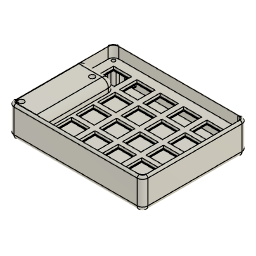
Diacritic Keypad (Autodesk Fusion 360 design; units mm, degrees)
Autodesk Fusion 360 part; units mm, degrees
sketch "Sketch1" plane through (0, 0, 0) normal (0, 0, 1) x (1, 0, 0)
  line L0 (-99.4421, 91.3159) -> (26.6579, 91.3159)
  line L1 (26.6579, 91.3159) -> (26.6579, -7.4341)
  line L2 (26.6579, -7.4341) -> (-99.4421, -7.4341)
  line L3 (-99.4421, -7.4341) -> (-99.4421, 91.3159)
  line L4 (-88.9421, 80.8159) -> (-71.8421, 80.8159)
  line L5 (-71.8421, 80.8159) -> (-71.8421, 64.5659)
  line L6 (-71.8421, 64.5659) -> (-88.9421, 64.5659)
  line L7 (-88.9421, 64.5659) -> (-88.9421, 80.8159)
  line L8 (-66.9421, 64.5659) -> (-66.9421, 80.8159)
  line L9 (-66.9421, 80.8159) -> (-49.8421, 80.8159)
  line L10 (-49.8421, 80.8159) -> (-49.8421, 64.5659)
  line L11 (-49.8421, 64.5659) -> (-66.9421, 64.5659)
  line L12 (-44.9421, 64.5659) -> (-44.9421, 80.8159)
  line L13 (-44.9421, 80.8159) -> (-27.8421, 80.8159)
  line L14 (-27.8421, 80.8159) -> (-27.8421, 64.5659)
  line L15 (-27.8421, 64.5659) -> (-44.9421, 64.5659)
  line L16 (-22.9421, 64.5659) -> (-22.9421, 80.8159)
  line L17 (-22.9421, 80.8159) -> (-5.8421, 80.8159)
  line L18 (-5.8421, 80.8159) -> (-5.8421, 64.5659)
  line L19 (-5.8421, 64.5659) -> (-22.9421, 64.5659)
  line L20 (-0.9421, 64.5659) -> (-0.9421, 80.8159)
  line L21 (-0.9421, 80.8159) -> (16.1579, 80.8159)
  line L22 (16.1579, 80.8159) -> (16.1579, 64.5659)
  line L23 (16.1579, 64.5659) -> (-0.9421, 64.5659)
  line L24 (-88.9421, 44.0659) -> (-88.9421, 60.3159)
  line L25 (-88.9421, 60.3159) -> (-71.8421, 60.3159)
  line L26 (-71.8421, 60.3159) -> (-71.8421, 44.0659)
  line L27 (-71.8421, 44.0659) -> (-88.9421, 44.0659)
  line L28 (-66.9421, 44.0659) -> (-66.9421, 60.3159)
  line L29 (-66.9421, 60.3159) -> (-49.8421, 60.3159)
  line L30 (-49.8421, 60.3159) -> (-49.8421, 44.0659)
  line L31 (-49.8421, 44.0659) -> (-66.9421, 44.0659)
  line L32 (-44.9421, 44.0659) -> (-44.9421, 60.3159)
  line L33 (-44.9421, 60.3159) -> (-27.8421, 60.3159)
  line L34 (-27.8421, 60.3159) -> (-27.8421, 44.0659)
  line L35 (-27.8421, 44.0659) -> (-44.9421, 44.0659)
  line L36 (-22.9421, 44.0659) -> (-22.9421, 60.3159)
  line L37 (-22.9421, 60.3159) -> (-5.8421, 60.3159)
  line L38 (-5.8421, 60.3159) -> (-5.8421, 44.0659)
  line L39 (-5.8421, 44.0659) -> (-22.9421, 44.0659)
  line L40 (-0.9421, 44.0659) -> (-0.9421, 60.3159)
  line L41 (-0.9421, 60.3159) -> (16.1579, 60.3159)
  line L42 (16.1579, 60.3159) -> (16.1579, 44.0659)
  line L43 (16.1579, 44.0659) -> (-0.9421, 44.0659)
  line L44 (-88.9421, 23.5659) -> (-88.9421, 39.8159)
  line L45 (-88.9421, 39.8159) -> (-71.8421, 39.8159)
  line L46 (-71.8421, 39.8159) -> (-71.8421, 23.5659)
  line L47 (-71.8421, 23.5659) -> (-88.9421, 23.5659)
  line L48 (-66.9421, 23.5659) -> (-66.9421, 39.8159)
  line L49 (-66.9421, 39.8159) -> (-49.8421, 39.8159)
  line L50 (-49.8421, 39.8159) -> (-49.8421, 23.5659)
  line L51 (-49.8421, 23.5659) -> (-66.9421, 23.5659)
  line L52 (-44.9421, 23.5659) -> (-44.9421, 39.8159)
  line L53 (-44.9421, 39.8159) -> (-27.8421, 39.8159)
  line L54 (-27.8421, 39.8159) -> (-27.8421, 23.5659)
  line L55 (-27.8421, 23.5659) -> (-44.9421, 23.5659)
  line L56 (-22.9421, 23.5659) -> (-22.9421, 39.8159)
  line L57 (-22.9421, 39.8159) -> (-5.8421, 39.8159)
  line L58 (-5.8421, 39.8159) -> (-5.8421, 23.5659)
  line L59 (-5.8421, 23.5659) -> (-22.9421, 23.5659)
  line L60 (-0.9421, 23.5659) -> (-0.9421, 39.8159)
  line L61 (-0.9421, 39.8159) -> (16.1579, 39.8159)
  line L62 (16.1579, 39.8159) -> (16.1579, 23.5659)
  line L63 (16.1579, 23.5659) -> (-0.9421, 23.5659)
  line L64 (-88.9421, 3.0659) -> (-88.9421, 19.3159)
  line L65 (-88.9421, 19.3159) -> (-71.8421, 19.3159)
  line L66 (-71.8421, 19.3159) -> (-71.8421, 3.0659)
  line L67 (-71.8421, 3.0659) -> (-88.9421, 3.0659)
  line L68 (-66.9421, 3.0659) -> (-66.9421, 19.3159)
  line L69 (-66.9421, 19.3159) -> (-49.8421, 19.3159)
  line L70 (-49.8421, 19.3159) -> (-49.8421, 3.0659)
  line L71 (-49.8421, 3.0659) -> (-66.9421, 3.0659)
  line L72 (-44.9421, 3.0659) -> (-44.9421, 19.3159)
  line L73 (-44.9421, 19.3159) -> (-27.8421, 19.3159)
  line L74 (-27.8421, 19.3159) -> (-27.8421, 3.0659)
  line L75 (-27.8421, 3.0659) -> (-44.9421, 3.0659)
  line L76 (-22.9421, 3.0659) -> (-22.9421, 19.3159)
  line L77 (-22.9421, 19.3159) -> (-5.8421, 19.3159)
  line L78 (-5.8421, 19.3159) -> (-5.8421, 3.0659)
  line L79 (-5.8421, 3.0659) -> (-22.9421, 3.0659)
  line L80 (-0.9421, 3.0659) -> (-0.9421, 19.3159)
  line L81 (-0.9421, 19.3159) -> (16.1579, 19.3159)
  line L82 (16.1579, 19.3159) -> (16.1579, 3.0659)
  line L83 (16.1579, 3.0659) -> (-0.9421, 3.0659)
  line L84 (-92.1145, 31.055) -> (-73.6145, 31.055)
  line L85 (-73.6145, 31.055) -> (-73.6145, -2.445)
  line L86 (-73.6145, -2.445) -> (-92.1145, -2.445)
  line L87 (-92.1145, -2.445) -> (-92.1145, 31.055)
  line L88 (24.6579, -5.4341) -> (-97.4421, -5.4341)
  line L89 (-97.4421, -5.4341) -> (-97.4421, 89.3159)
  line L90 (-97.4421, 89.3159) -> (24.6579, 89.3159)
  line L91 (24.6579, 89.3159) -> (24.6579, -5.4341)
  line L92 (-97.4421, 89.3159) -> (-89.4421, 89.3159)
  line L93 (-89.4421, 89.3159) -> (-89.4421, 81.3159)
  line L94 (-89.4421, 81.3159) -> (-97.4421, 81.3159)
  line L95 (-97.4421, 81.3159) -> (-97.4421, 89.3159)
  line L96 (24.6579, 89.3159) -> (16.6579, 89.3159)
  line L97 (16.6579, 89.3159) -> (16.6579, 81.3159)
  line L98 (16.6579, 81.3159) -> (24.6579, 81.3159)
  line L99 (24.6579, 81.3159) -> (24.6579, 89.3159)
  line L100 (24.6579, -5.4341) -> (16.6579, -5.4341)
  line L101 (16.6579, -5.4341) -> (16.6579, 2.5659)
  line L102 (16.6579, 2.5659) -> (24.6579, 2.5659)
  line L103 (24.6579, 2.5659) -> (24.6579, -5.4341)
  line L104 (-97.4421, -5.4341) -> (-89.4421, -5.4341)
  line L105 (-89.4421, -5.4341) -> (-89.4421, 2.5659)
  line L106 (-89.4421, 2.5659) -> (-97.4421, 2.5659)
  line L107 (-97.4421, 2.5659) -> (-97.4421, -5.4341)
  line L108 (-69.3921, 62.4409) -> (-97.4421, 62.4409)
  line L109 (-97.4421, 62.4409) -> (-97.4421, -5.4341)
  line L110 (-97.4421, -5.4341) -> (-69.3921, -5.4341)
  line L111 (-69.3921, -5.4341) -> (-69.3921, 62.4409)
  line L112 (-71.8421, 32.9465) -> (-69.3921, 32.9465) construction
  line L113 (-66.9421, 32.9465) -> (-69.3921, 32.9465) construction
  line L114 (-97.4421, 89.3159) -> (-89.4421, 81.3159) construction
  circle A0 centre (-93.4421, 85.3159) radius 2.125
  line L115 (16.6579, 81.3159) -> (24.6579, 89.3159) construction
  circle A1 centre (20.6579, 85.3159) radius 2.125
  line L116 (16.6579, 2.5659) -> (24.6579, -5.4341) construction
  line L117 (-89.4421, 2.5659) -> (-97.4421, -5.4341) construction
  circle A2 centre (-93.4421, -1.4341) radius 2.125
  circle A3 centre (20.6579, -1.4341) radius 2.125
  line L118 (-79.8732, 60.3159) -> (-79.8732, 62.4409) construction
  line L119 (-79.8732, 62.4409) -> (-79.8732, 64.5659) construction
  circle A4 centre (-93.4421, 85.3159) radius 1.625
  circle A5 centre (20.6579, 85.3159) radius 1.625
  circle A6 centre (20.6579, -1.4341) radius 1.625
  circle A7 centre (-93.4421, -1.4341) radius 1.625
  circle A8 centre (-93.4421, -1.4341) radius 2.5
  dimension "d1" = 17.1
  dimension "d2" = 16.25
  dimension "d6" = 88
  dimension "d7" = -61.5
  dimension "d8" = 4.9
  dimension "d9" = 4.25
  dimension "d10" = 10.5
  dimension "d11" = 10.5
  dimension "d12" = 10.5
  dimension "d13" = 10.5
  dimension "d14" = 18.5
  dimension "d15" = 33.5
  dimension "d16" = 2
  dimension "d21" = 8
  dimension "d22" = 8
  dimension "d23" = 8
  dimension "d24" = 8
  dimension "d25" = 8
  dimension "d26" = 8
  dimension "d27" = 8
  dimension "d28" = 8
  dimension "d76" = 4.25
  dimension "d77" = 4.25
  dimension "d78" = 4.25
  dimension "d79" = 4.25
  dimension "d106" = 3.25
  dimension "d107" = 3.25
  dimension "d108" = 3.25
  dimension "d109" = 3.25
  dimension "d112" = 5
  constraint horizontal L0
  constraint vertical L1
  constraint horizontal L2
  constraint vertical L3
  constraint horizontal L4
  constraint vertical L5
  constraint horizontal L6
  constraint vertical L7
  constraint horizontal L84
  constraint vertical L85
  constraint horizontal L86
  constraint vertical L87
  constraint horizontal L92
  constraint vertical L93
  constraint horizontal L94
  constraint vertical L95
  constraint horizontal L96
  constraint vertical L97
  constraint horizontal L98
  constraint vertical L99
  constraint horizontal L100
  constraint vertical L101
  constraint horizontal L102
  constraint vertical L103
  constraint horizontal L104
  constraint vertical L105
  constraint horizontal L106
  constraint vertical L107
  constraint horizontal L108
  constraint vertical L109
  constraint horizontal L110
  constraint vertical L111
  constraint coincident L46 L112.start
  constraint coincident L111 L112.end
  constraint perpendicular L111 L112
  constraint coincident L48 L113.start
  constraint perpendicular L111 L113
  constraint equal L112 L113
  constraint midpoint L114 A0.centre
  constraint midpoint L115 A1.centre
  constraint midpoint L117 A2.centre
  constraint midpoint L116 A3.centre
  constraint coincident L25 L118.start
  constraint coincident L108 L118.end
  constraint perpendicular L108 L118
  constraint coincident L6 L119.end
  constraint perpendicular L6 L119
  constraint equal L118 L119
  constraint concentric A0 A4
  constraint concentric A1 A5
  constraint concentric A3 A6
  constraint concentric A2 A7
  constraint concentric A2 A8
  measures "d1" distance of L4.start L4.end
  measures "d2" distance of L4.start L6.end
  measures "d8" distance of L5 L8
  measures "d9" distance of L6 L25
  measures "d10" distance of L0 L4
  measures "d11" distance of L3 L7
  measures "d12" distance of L1 L22
  measures "d13" distance of L2 L83
  measures "d14" distance of L84.start L84.end
  measures "d15" distance of L84.start L86.end
  measures "d21" distance of L89.end L92.end
  measures "d22" distance of L89.end L94.end
  measures "d23" distance of L90.end L96.end
  measures "d24" distance of L90.end L98.end
  measures "d25" distance of L88.start L100.end
  measures "d26" distance of L88.start L102.end
  measures "d27" distance of L88.end L104.end
  measures "d28" distance of L88.end L106.end
  measures "d76" diameter of A0
  measures "d77" diameter of A1
  measures "d78" diameter of A2
  measures "d79" diameter of A3
  measures "d106" diameter of A4
  measures "d107" diameter of A5
  measures "d108" diameter of A6
  measures "d109" diameter of A7
  measures "d112" diameter of A8
extrude "Extrude1" add sketch "Sketch1" against normal blind 2 contours L0 L1 L2 L3 | L4 L5 L6 L7 | L8 L9 L10 L11 | L12 L13 L14 L15 | L16 L17 L18 L19 | L20 L21 L22 L23 | L24 L25 L26 L27 | L28 L29 L30 L31 | L32 L33 L34 L35 | L36 L37 L38 L39 | L40 L41 L42 L43 | L44 L47 L64 L65 L67 L84 L85 L86 L87 L105 L106 | L44 L47 L84 L85 | L44 L45 L46 L47 L65 L66 L67 L84 L85 L86 L87 L88 L89 L105 L106 L108 L109 L110 L111 | L44 L45 L46 L47 L84 L85 | L64 L65 L67 L85 | L65 L66 L67 L85 | L86 L87 L105 L106 A8 | L86 L87 L88 L89 L104 L105 L106 L107 L109 L110 A8 | L86 L87 A2 A8 | L86 L87 A2 A8 | L86 L87 A2 A7 | L86 L87 A2 A7 | L88 L89 L90 L91 L93 L94 L97 L98 L101 L102 L108 L111 | L87 A7 | L87 A7 | L89 L90 L92 L93 L94 L95 | L88 L91 L100 L101 L102 L103 | L90 L91 L96 L97 L98 L99 | L48 L49 L50 L51 | L52 L53 L54 L55 | L56 L57 L58 L59 | L60 L61 L62 L63 | L68 L69 L70 L71 | L72 L73 L74 L75 | L76 L77 L78 L79 | L80 L81 L82 L83 | A0 | A1 | A3 | A4 | A5 | A6 makes body 1
extrude "Extrude2" add sketch "Sketch1" along normal blind 28 contours L0 L1 L2 L3 bodies 1
extrude "Extrude3" add sketch "Sketch1" along normal blind 14.5 contours L86 L87 L105 L106 A8 | L86 L87 L88 L89 L104 L105 L106 L107 L109 L110 A8 | L86 L87 A2 A8 | L86 L87 A2 A8 | L89 L90 L92 L93 L94 L95 | L88 L91 L100 L101 L102 L103 | L90 L91 L96 L97 L98 L99 bodies 1
extrude "Extrude4" add sketch "Sketch1" along normal blind 2.5 from surface at 14.5 separate body contours L44 L47 L64 L65 L67 L84 L85 L86 L87 L105 L106 | L44 L47 L84 L85 | L44 L45 L46 L47 L65 L66 L67 L84 L85 L86 L87 L88 L89 L105 L106 L108 L109 L110 L111 | L44 L45 L46 L47 L84 L85 | L64 L65 L67 L85 | L65 L66 L67 L85 | L86 L87 L105 L106 A8 | L86 L87 L88 L89 L104 L105 L106 L107 L109 L110 A8 | L86 L87 A2 A8 | L86 L87 A2 A8 | L86 L87 A2 A7 | L86 L87 A2 A7 | L88 L89 L90 L91 L93 L94 L97 L98 L101 L102 L108 L111 | L87 A7 | L87 A7 | L89 L90 L92 L93 L94 L95 | L88 L91 L100 L101 L102 L103 | L90 L91 L96 L97 L98 L99 | A0 | A1 | A3 | A4 | A5 | A6 makes body 2
extrude "Extrude5" cut 1 faces at (-16.0421, -6.7674, 28) along direction (0, 0, -1) blind 0.4 on bodies 1 bodies 1
extrude "Extrude7" add sketch "Sketch1" along normal blind 10 from surface at 17 contours L24 L25 L26 L27 | L44 L47 L64 L65 L67 L84 L85 L86 L87 L105 L106 | L44 L47 L84 L85 | L44 L45 L46 L47 L65 L66 L67 L84 L85 L86 L87 L88 L89 L105 L106 L108 L109 L110 L111 | L44 L45 L46 L47 L84 L85 | L64 L65 L67 L85 | L65 L66 L67 L85 | L86 L87 L105 L106 A8 | L86 L87 L88 L89 L104 L105 L106 L107 L109 L110 A8 | L86 L87 A2 A8 | L86 L87 A2 A8 | L86 L87 A2 A7 | L86 L87 A2 A7 | L87 A7 | L87 A7 bodies 2
extrude "Extrude8" cut 1 faces at (-88.0921, -5.4341, 19.5) along direction (0, 1, 0) blind 0.3 on bodies 2 bodies 2
extrude "Extrude9" cut 1 faces at (24.6579, 57.8326, 15.3333) along direction (-1, 0, 0) blind 0.3 on bodies 2 bodies 2
extrude "Extrude10" cut 1 faces at (-56.8421, 89.3159, 15.3333) along direction (0, -1, 0) blind 0.3 on bodies 2 bodies 2
extrude "Extrude11" cut 1 faces at (-97.4421, 17.3909, 19.5) along direction (1, 0, 0) blind 0.3 on bodies 2 bodies 2
extrude "Extrude19" cut sketch "Sketch1" along normal blind 18 contours L87 A7 | L87 A7 | A4 | A5 | A6 bodies 2
extrude "Extrude20" cut sketch "Sketch1" along normal blind 15.5 from surface at 18 contours L86 L87 A2 A8 | L86 L87 A2 A8 | L86 L87 A2 A7 | L86 L87 A2 A7 | L87 A7 | L87 A7 bodies 2
fillet "Fillet1" radius 5 12 edges at (-99.4421, -7.4341, 12.8) (-99.4421, 91.3159, 12.8) (26.6579, 91.3159, 12.8) (26.6579, -7.4341, 12.8) (24.6579, -5.4341, 21.05) (-97.4421, -5.4341, 21.05) (-97.4421, 89.3159, 21.05) (24.6579, 89.3159, 21.05) (-97.1421, -5.1341, 20.75) (-97.1421, 89.0159, 15.75) (24.3579, 89.0159, 15.75) (24.3579, -5.1341, 15.75) on bodies 1 2
fillet "Fillet2" radius 5 8 edges at (25.1934, -5.9696, -2) (-36.3921, -7.4341, -2) (-97.9776, -5.9696, -2) (-99.4421, 41.9409, -2) (-97.9776, 89.8515, -2) (-36.3921, 91.3159, -2) (25.1934, 89.8515, -2) (26.6579, 41.9409, -2) on bodies 1
fillet "Fillet3" radius 2 8 edges at (-36.3921, 91.3159, 27.6) (25.1934, 89.8515, 27.6) (26.6579, 41.9409, 27.6) (25.1934, -5.9696, 27.6) (-36.3921, -7.4341, 27.6) (-97.9776, -5.9696, 27.6) (-99.4421, 41.9409, 27.6) (-97.9776, 89.8515, 27.6) on bodies 1
fillet "Fillet4" radius 6 3 edges at (-83.2671, 62.4409, 27) (-69.3921, 28.6534, 27) (-69.3921, 62.4409, 22) on bodies 2
fillet "Fillet5" radius 2.5 12 edges at (-97.4421, 81.3159, 7.25) (-89.4421, 81.3159, 7.25) (-89.4421, 89.3159, 7.25) (16.6579, 89.3159, 7.25) (16.6579, 81.3159, 7.25) (24.6579, 81.3159, 7.25) (-89.4421, -5.4341, 7.25) (-89.4421, 2.5659, 7.25) (-97.4421, 2.5659, 7.25) (16.6579, -5.4341, 7.25) (16.6579, 2.5659, 7.25) (24.6579, 2.5659, 7.25) on bodies 1
extrude "Extrude12" add 4 faces at (-94, -2.432, 0) (21.3662, 84.3524, 0) (20.0197, -1.7414, 0) (-92.5065, 85.7665, 0) along direction (0, 0, 1) blind 4 on bodies 1 bodies 1
sketch "Sketch2" plane through (0, 0, 14.5) normal (0, 0, -1) x (1, 0, 0)
  line L0 (-27.8421, -19.3159) -> (-44.9421, -19.3159)
  line L1 (-44.9421, -19.3159) -> (-44.9421, -3.0659)
  line L2 (-44.9421, -3.0659) -> (-27.8421, -3.0659)
  line L3 (-27.8421, -3.0659) -> (-27.8421, -19.3159)
  line L4 (-5.8421, -19.3159) -> (-22.9421, -19.3159)
  line L5 (-22.9421, -19.3159) -> (-22.9421, -3.0659)
  line L6 (-22.9421, -3.0659) -> (-5.8421, -3.0659)
  line L7 (-5.8421, -3.0659) -> (-5.8421, -19.3159)
  line L8 (16.1579, -19.3159) -> (-0.9421, -19.3159)
  line L9 (-0.9421, -19.3159) -> (-0.9421, -3.0659)
  line L10 (-0.9421, -3.0659) -> (16.1579, -3.0659)
  line L11 (16.1579, -3.0659) -> (16.1579, -19.3159)
  line L12 (-71.8421, -64.5659) -> (-71.8421, -80.8159)
  line L13 (-71.8421, -80.8159) -> (-88.9421, -80.8159)
  line L14 (-88.9421, -80.8159) -> (-88.9421, -64.5659)
  line L15 (-88.9421, -64.5659) -> (-71.8421, -64.5659)
  line L16 (-49.8421, -80.8159) -> (-66.9421, -80.8159)
  line L17 (-66.9421, -80.8159) -> (-66.9421, -64.5659)
  line L18 (-66.9421, -64.5659) -> (-49.8421, -64.5659)
  line L19 (-49.8421, -64.5659) -> (-49.8421, -80.8159)
  line L20 (-5.8421, -80.8159) -> (-22.9421, -80.8159)
  line L21 (-22.9421, -80.8159) -> (-22.9421, -64.5659)
  line L22 (-22.9421, -64.5659) -> (-5.8421, -64.5659)
  line L23 (-5.8421, -64.5659) -> (-5.8421, -80.8159)
  line L24 (-27.8421, -80.8159) -> (-44.9421, -80.8159)
  line L25 (-44.9421, -80.8159) -> (-44.9421, -64.5659)
  line L26 (-44.9421, -64.5659) -> (-27.8421, -64.5659)
  line L27 (-27.8421, -64.5659) -> (-27.8421, -80.8159)
  line L28 (-49.8421, -39.8159) -> (-66.9421, -39.8159)
  line L29 (-66.9421, -39.8159) -> (-66.9421, -23.5659)
  line L30 (-66.9421, -23.5659) -> (-49.8421, -23.5659)
  line L31 (-49.8421, -23.5659) -> (-49.8421, -39.8159)
  line L32 (-5.8421, -60.3159) -> (-22.9421, -60.3159)
  line L33 (-22.9421, -60.3159) -> (-22.9421, -44.0659)
  line L34 (-22.9421, -44.0659) -> (-5.8421, -44.0659)
  line L35 (-5.8421, -44.0659) -> (-5.8421, -60.3159)
  line L36 (-49.8421, -60.3159) -> (-66.9421, -60.3159)
  line L37 (-66.9421, -60.3159) -> (-66.9421, -44.0659)
  line L38 (-66.9421, -44.0659) -> (-49.8421, -44.0659)
  line L39 (-49.8421, -44.0659) -> (-49.8421, -60.3159)
  line L40 (16.1579, -39.8159) -> (-0.9421, -39.8159)
  line L41 (-0.9421, -39.8159) -> (-0.9421, -23.5659)
  line L42 (-0.9421, -23.5659) -> (16.1579, -23.5659)
  line L43 (16.1579, -23.5659) -> (16.1579, -39.8159)
  line L44 (-49.8421, -19.3159) -> (-66.9421, -19.3159)
  line L45 (-66.9421, -19.3159) -> (-66.9421, -3.0659)
  line L46 (-66.9421, -3.0659) -> (-49.8421, -3.0659)
  line L47 (-49.8421, -3.0659) -> (-49.8421, -19.3159)
  line L48 (-5.8421, -39.8159) -> (-22.9421, -39.8159)
  line L49 (-22.9421, -39.8159) -> (-22.9421, -23.5659)
  line L50 (-22.9421, -23.5659) -> (-5.8421, -23.5659)
  line L51 (-5.8421, -23.5659) -> (-5.8421, -39.8159)
  line L52 (-27.8421, -60.3159) -> (-44.9421, -60.3159)
  line L53 (-44.9421, -60.3159) -> (-44.9421, -44.0659)
  line L54 (-44.9421, -44.0659) -> (-27.8421, -44.0659)
  line L55 (-27.8421, -44.0659) -> (-27.8421, -60.3159)
  line L56 (-71.8421, -60.3159) -> (-88.9421, -60.3159)
  line L57 (-88.9421, -60.3159) -> (-88.9421, -44.0659)
  line L58 (-88.9421, -44.0659) -> (-71.8421, -44.0659)
  line L59 (-71.8421, -44.0659) -> (-71.8421, -60.3159)
  line L60 (-27.8421, -39.8159) -> (-44.9421, -39.8159)
  line L61 (-44.9421, -39.8159) -> (-44.9421, -23.5659)
  line L62 (-44.9421, -23.5659) -> (-27.8421, -23.5659)
  line L63 (-27.8421, -23.5659) -> (-27.8421, -39.8159)
  line L64 (16.1579, -80.8159) -> (-0.9421, -80.8159)
  line L65 (-0.9421, -80.8159) -> (-0.9421, -64.5659)
  line L66 (-0.9421, -64.5659) -> (16.1579, -64.5659)
  line L67 (16.1579, -64.5659) -> (16.1579, -80.8159)
  line L68 (16.1579, -60.3159) -> (-0.9421, -60.3159)
  line L69 (-0.9421, -60.3159) -> (-0.9421, -44.0659)
  line L70 (-0.9421, -44.0659) -> (16.1579, -44.0659)
  line L71 (16.1579, -44.0659) -> (16.1579, -60.3159)
  line L72 (-50.4671, -18.6909) -> (-66.3171, -18.6909)
  line L73 (-66.3171, -18.6909) -> (-66.3171, -3.6909)
  line L74 (-66.3171, -3.6909) -> (-50.4671, -3.6909)
  line L75 (-50.4671, -3.6909) -> (-50.4671, -18.6909)
  line L76 (-28.4671, -3.6909) -> (-28.4671, -18.6909)
  line L77 (-28.4671, -18.6909) -> (-44.3171, -18.6909)
  line L78 (-44.3171, -18.6909) -> (-44.3171, -3.6909)
  line L79 (-44.3171, -3.6909) -> (-28.4671, -3.6909)
  line L80 (-6.4671, -18.6909) -> (-22.3171, -18.6909)
  line L81 (-22.3171, -18.6909) -> (-22.3171, -3.6909)
  line L82 (-22.3171, -3.6909) -> (-6.4671, -3.6909)
  line L83 (-6.4671, -3.6909) -> (-6.4671, -18.6909)
  line L84 (-0.3171, -3.6909) -> (15.5329, -3.6909)
  line L85 (15.5329, -3.6909) -> (15.5329, -18.6909)
  line L86 (15.5329, -18.6909) -> (-0.3171, -18.6909)
  line L87 (-0.3171, -18.6909) -> (-0.3171, -3.6909)
  line L88 (-50.4671, -39.1909) -> (-66.3171, -39.1909)
  line L89 (-66.3171, -39.1909) -> (-66.3171, -24.1909)
  line L90 (-66.3171, -24.1909) -> (-50.4671, -24.1909)
  line L91 (-50.4671, -24.1909) -> (-50.4671, -39.1909)
  line L92 (-28.4671, -24.1909) -> (-28.4671, -39.1909)
  line L93 (-28.4671, -39.1909) -> (-44.3171, -39.1909)
  line L94 (-44.3171, -39.1909) -> (-44.3171, -24.1909)
  line L95 (-44.3171, -24.1909) -> (-28.4671, -24.1909)
  line L96 (-6.4671, -39.1909) -> (-22.3171, -39.1909)
  line L97 (-22.3171, -39.1909) -> (-22.3171, -24.1909)
  line L98 (-22.3171, -24.1909) -> (-6.4671, -24.1909)
  line L99 (-6.4671, -24.1909) -> (-6.4671, -39.1909)
  line L100 (15.5329, -39.1909) -> (-0.3171, -39.1909)
  line L101 (-0.3171, -39.1909) -> (-0.3171, -24.1909)
  line L102 (-0.3171, -24.1909) -> (15.5329, -24.1909)
  line L103 (15.5329, -24.1909) -> (15.5329, -39.1909)
  line L104 (15.5329, -44.6909) -> (15.5329, -59.6909)
  line L105 (15.5329, -59.6909) -> (-0.3171, -59.6909)
  line L106 (-0.3171, -59.6909) -> (-0.3171, -44.6909)
  line L107 (-0.3171, -44.6909) -> (15.5329, -44.6909)
  line L108 (-6.4671, -59.6909) -> (-22.3171, -59.6909)
  line L109 (-22.3171, -59.6909) -> (-22.3171, -44.6909)
  line L110 (-22.3171, -44.6909) -> (-6.4671, -44.6909)
  line L111 (-6.4671, -44.6909) -> (-6.4671, -59.6909)
  line L112 (-44.3171, -59.6909) -> (-44.3171, -44.6909)
  line L113 (-44.3171, -44.6909) -> (-28.4671, -44.6909)
  line L114 (-28.4671, -44.6909) -> (-28.4671, -59.6909)
  line L115 (-28.4671, -59.6909) -> (-44.3171, -59.6909)
  line L116 (-66.3171, -59.6909) -> (-66.3171, -44.6909)
  line L117 (-66.3171, -44.6909) -> (-50.4671, -44.6909)
  line L118 (-50.4671, -44.6909) -> (-50.4671, -59.6909)
  line L119 (-50.4671, -59.6909) -> (-66.3171, -59.6909)
  line L120 (-88.3171, -59.6909) -> (-88.3171, -44.6909)
  line L121 (-88.3171, -44.6909) -> (-72.4671, -44.6909)
  line L122 (-72.4671, -44.6909) -> (-72.4671, -59.6909)
  line L123 (-72.4671, -59.6909) -> (-88.3171, -59.6909)
  line L124 (-88.3171, -80.1909) -> (-88.3171, -65.1909)
  line L125 (-88.3171, -65.1909) -> (-72.4671, -65.1909)
  line L126 (-72.4671, -65.1909) -> (-72.4671, -80.1909)
  line L127 (-72.4671, -80.1909) -> (-88.3171, -80.1909)
  line L128 (-50.4671, -65.1909) -> (-50.4671, -80.1909)
  line L129 (-50.4671, -80.1909) -> (-66.3171, -80.1909)
  line L130 (-66.3171, -80.1909) -> (-66.3171, -65.1909)
  line L131 (-66.3171, -65.1909) -> (-50.4671, -65.1909)
  line L132 (-28.4671, -65.1909) -> (-28.4671, -80.1909)
  line L133 (-28.4671, -80.1909) -> (-44.3171, -80.1909)
  line L134 (-44.3171, -80.1909) -> (-44.3171, -65.1909)
  line L135 (-44.3171, -65.1909) -> (-28.4671, -65.1909)
  line L136 (-6.4671, -80.1909) -> (-22.3171, -80.1909)
  line L137 (-22.3171, -80.1909) -> (-22.3171, -65.1909)
  line L138 (-22.3171, -65.1909) -> (-6.4671, -65.1909)
  line L139 (-6.4671, -65.1909) -> (-6.4671, -80.1909)
  line L140 (15.5329, -65.1909) -> (15.5329, -80.1909)
  line L141 (15.5329, -80.1909) -> (-0.3171, -80.1909)
  line L142 (-0.3171, -80.1909) -> (-0.3171, -65.1909)
  line L143 (-0.3171, -65.1909) -> (15.5329, -65.1909)
  arc A0 (24.3579, 0.1341) -> (19.3579, 5.1341) centre (19.3579, 0.1341) ccw
  line L144 (19.3579, 5.1341) -> (-92.1421, 5.1341)
  arc A1 (-92.1421, 5.1341) -> (-97.1421, 0.1341) centre (-92.1421, 0.1341) ccw
  line L145 (-97.1421, 0.1341) -> (-97.1421, -84.0159)
  arc A2 (-97.1421, -84.0159) -> (-92.1421, -89.0159) centre (-92.1421, -84.0159) ccw
  line L146 (-92.1421, -89.0159) -> (19.3579, -89.0159)
  arc A3 (19.3579, -89.0159) -> (24.3579, -84.0159) centre (19.3579, -84.0159) ccw
  line L147 (24.3579, -84.0159) -> (24.3579, 0.1341)
  circle A4 centre (-93.4421, 1.4341) radius 1.625
  circle A5 centre (-93.4421, -85.3159) radius 1.625
  circle A6 centre (20.6579, 1.4341) radius 1.625
  circle A7 centre (20.6579, -85.3159) radius 1.625
  dimension "d36" = 0.625
  dimension "d37" = 0.625
  dimension "d39" = 0.625
  dimension "d40" = 0.625
  dimension "d41" = 0.625
  dimension "d42" = 0.625
  dimension "d43" = 0.625
  dimension "d44" = 0.625
  dimension "d45" = 0.625
  dimension "d46" = 0.625
  dimension "d47" = 0.625
  dimension "d48" = 0.625
  dimension "d49" = 0.625
  dimension "d50" = 0.625
  dimension "d51" = 0.625
  dimension "d52" = 0.625
  dimension "d53" = 0.625
  dimension "d54" = 0.625
extrude "Extrude6" add sketch "Sketch2" along normal blind 0.6 contours L0 L1 L2 L3 | L4 L5 L6 L7 | L8 L9 L10 L11 | L12 L13 L14 L15 | L16 L17 L18 L19 | L20 L21 L22 L23 | L24 L25 L26 L27 | L28 L29 L30 L31 | L32 L33 L34 L35 | L36 L37 L38 L39 | L40 L41 L42 L43 | L44 L45 L46 L47 | L48 L49 L50 L51 | L52 L53 L54 L55 | L56 L57 L58 L59 | L60 L61 L62 L63 | L64 L65 L66 L67 | L68 L69 L70 L71 | A0 L144 A1 L145 A2 L146 A3 L147 bodies 2
move_body "Move1" bodies 2 to x (1, 0, 0) y (0, 1, 0) z (0, 0, 1) at (0, 0, 0.6)
extrude "Extrude13" add 1 faces at (-77.5421, 49.4826, 17.6) along direction (0, 0, -1) blind 3.1 on bodies 2 bodies 2
sketch "Sketch3" plane through (-97.4421, 0, 0) normal (1, 0, 0) x (0, 1, 0)
  line L0 (5.0659, 14.5) -> (5.0659, 0)
  line L1 (5.0659, 0) -> (78.8159, 0)
  line L2 (78.8159, 0) -> (78.8159, 14.5)
  line L3 (78.8159, 14.5) -> (84.3159, 14.5)
  line L4 (84.3159, 14.5) -> (84.3159, 27.6)
  line L5 (84.3159, 27.6) -> (-0.4341, 27.6)
  line L6 (-0.4341, 27.6) -> (-0.4341, 14.5)
  line L7 (-0.4341, 14.5) -> (5.0659, 14.5)
  line L8 (55.3537, 12.9074) -> (76.1037, 12.9074)
  line L9 (76.1037, 12.9074) -> (76.1037, 1.0574)
  line L10 (76.1037, 1.0574) -> (55.3537, 1.0574)
  line L11 (55.3537, 1.0574) -> (55.3537, 12.9074)
  dimension "d86" = 20.75
  dimension "d87" = 11.85
  constraint horizontal L8
  constraint vertical L9
  constraint horizontal L10
  constraint vertical L11
  measures "d86" distance of L8.start L8.end
  measures "d87" distance of L8.start L10.end
extrude "Extrude14" cut sketch "Sketch3" against normal blind 5 contours L8 L9 L10 L11 bodies 1
sketch "Sketch4" plane through (0, 89.3159, 0) normal (0, -1, 0) x (1, 0, 0)
  line L0 (14.1579, 0) -> (14.1579, 14.5)
  line L1 (14.1579, 14.5) -> (19.6579, 14.5)
  line L2 (19.6579, 14.5) -> (19.6579, 27.6)
  line L3 (19.6579, 27.6) -> (-92.4421, 27.6)
  line L4 (-92.4421, 27.6) -> (-92.4421, 14.5)
  line L5 (-92.4421, 14.5) -> (-86.9421, 14.5)
  line L6 (-86.9421, 14.5) -> (-86.9421, 0)
  line L7 (-86.9421, 0) -> (14.1579, 0)
  line L8 (-86.5962, 7.1262) -> (-76.0962, 7.1262)
  line L9 (-76.0962, 7.1262) -> (-76.0962, 1.1262)
  line L10 (-76.0962, 1.1262) -> (-86.5962, 1.1262)
  line L11 (-86.5962, 1.1262) -> (-86.5962, 7.1262)
  dimension "d90" = 10.5
  dimension "d91" = 6
  constraint horizontal L8
  constraint vertical L9
  constraint horizontal L10
  constraint vertical L11
  measures "d90" distance of L8.start L8.end
  measures "d91" distance of L8.start L10.end
extrude "Extrude15" cut sketch "Sketch4" against normal blind 7 contours L8 L9 L10 L11 bodies 1
fillet "Fillet6" radius 2.25 4 edges at (-76.0962, 90.1337, 1.1262) (-76.0962, 90.3159, 7.1262) (-86.5962, 90.3159, 7.1262) (-86.5962, 90.1337, 1.1262) on bodies 1
sketch "Sketch5" plane through (0, 0, 27.6) normal (0, 0, 1) x (-1, 0, 0)
  line L0 (75.3921, -56.4409) -> (97.1421, -56.4409)
  line L1 (97.1421, -56.4409) -> (97.1421, 0.1341)
  arc A0 (97.1421, 0.1341) -> (92.1421, 5.1341) centre (92.1421, 0.1341) ccw
  line L2 (92.1421, 5.1341) -> (75.3921, 5.1341)
  line L3 (75.3921, 5.1341) -> (75.3921, -56.4409)
  circle A1 centre (80.3921, -52.1909) radius 2.425
  circle A2 centre (80.3921, -52.1909) radius 3.125
  line L4 (22.9421, -60.3159) -> (5.8421, -60.3159)
  line L5 (5.8421, -60.3159) -> (5.8421, -44.0659)
  line L6 (5.8421, -44.0659) -> (22.9421, -44.0659)
  line L7 (22.9421, -44.0659) -> (22.9421, -60.3159)
  line L8 (44.9421, -60.3159) -> (27.8421, -60.3159)
  line L9 (27.8421, -60.3159) -> (27.8421, -44.0659)
  line L10 (27.8421, -44.0659) -> (44.9421, -44.0659)
  line L11 (44.9421, -44.0659) -> (44.9421, -60.3159)
  line L12 (66.9421, -60.3159) -> (49.8421, -60.3159)
  line L13 (49.8421, -60.3159) -> (49.8421, -44.0659)
  line L14 (49.8421, -44.0659) -> (66.9421, -44.0659)
  line L15 (66.9421, -44.0659) -> (66.9421, -60.3159)
  line L16 (0.9421, -80.8159) -> (-16.1579, -80.8159)
  line L17 (-16.1579, -80.8159) -> (-16.1579, -64.5659)
  line L18 (-16.1579, -64.5659) -> (0.9421, -64.5659)
  line L19 (0.9421, -64.5659) -> (0.9421, -80.8159)
  line L20 (66.9421, -39.8159) -> (49.8421, -39.8159)
  line L21 (49.8421, -39.8159) -> (49.8421, -23.5659)
  line L22 (49.8421, -23.5659) -> (66.9421, -23.5659)
  line L23 (66.9421, -23.5659) -> (66.9421, -39.8159)
  line L24 (44.9421, -39.8159) -> (27.8421, -39.8159)
  line L25 (27.8421, -39.8159) -> (27.8421, -23.5659)
  line L26 (27.8421, -23.5659) -> (44.9421, -23.5659)
  line L27 (44.9421, -23.5659) -> (44.9421, -39.8159)
  line L28 (0.9421, -60.3159) -> (-16.1579, -60.3159)
  line L29 (-16.1579, -60.3159) -> (-16.1579, -44.0659)
  line L30 (-16.1579, -44.0659) -> (0.9421, -44.0659)
  line L31 (0.9421, -44.0659) -> (0.9421, -60.3159)
  line L32 (22.9421, -39.8159) -> (5.8421, -39.8159)
  line L33 (5.8421, -39.8159) -> (5.8421, -23.5659)
  line L34 (5.8421, -23.5659) -> (22.9421, -23.5659)
  line L35 (22.9421, -23.5659) -> (22.9421, -39.8159)
  line L36 (0.9421, -39.8159) -> (-16.1579, -39.8159)
  line L37 (-16.1579, -39.8159) -> (-16.1579, -23.5659)
  line L38 (-16.1579, -23.5659) -> (0.9421, -23.5659)
  line L39 (0.9421, -23.5659) -> (0.9421, -39.8159)
  line L40 (66.9421, -19.3159) -> (49.8421, -19.3159)
  line L41 (49.8421, -19.3159) -> (49.8421, -3.0659)
  line L42 (49.8421, -3.0659) -> (66.9421, -3.0659)
  line L43 (66.9421, -3.0659) -> (66.9421, -19.3159)
  line L44 (44.9421, -19.3159) -> (27.8421, -19.3159)
  line L45 (27.8421, -19.3159) -> (27.8421, -3.0659)
  line L46 (27.8421, -3.0659) -> (44.9421, -3.0659)
  line L47 (44.9421, -3.0659) -> (44.9421, -19.3159)
  line L48 (22.9421, -19.3159) -> (5.8421, -19.3159)
  line L49 (5.8421, -19.3159) -> (5.8421, -3.0659)
  line L50 (5.8421, -3.0659) -> (22.9421, -3.0659)
  line L51 (22.9421, -3.0659) -> (22.9421, -19.3159)
  line L52 (0.9421, -19.3159) -> (-16.1579, -19.3159)
  line L53 (-16.1579, -19.3159) -> (-16.1579, -3.0659)
  line L54 (-16.1579, -3.0659) -> (0.9421, -3.0659)
  line L55 (0.9421, -3.0659) -> (0.9421, -19.3159)
  line L56 (71.8421, -80.8159) -> (71.8421, -64.5659)
  line L57 (71.8421, -64.5659) -> (88.9421, -64.5659)
  line L58 (88.9421, -64.5659) -> (88.9421, -80.8159)
  line L59 (88.9421, -80.8159) -> (71.8421, -80.8159)
  line L60 (66.9421, -80.8159) -> (49.8421, -80.8159)
  line L61 (49.8421, -80.8159) -> (49.8421, -64.5659)
  line L62 (49.8421, -64.5659) -> (66.9421, -64.5659)
  line L63 (66.9421, -64.5659) -> (66.9421, -80.8159)
  line L64 (22.9421, -80.8159) -> (5.8421, -80.8159)
  line L65 (5.8421, -80.8159) -> (5.8421, -64.5659)
  line L66 (5.8421, -64.5659) -> (22.9421, -64.5659)
  line L67 (22.9421, -64.5659) -> (22.9421, -80.8159)
  line L68 (44.9421, -80.8159) -> (27.8421, -80.8159)
  line L69 (27.8421, -80.8159) -> (27.8421, -64.5659)
  line L70 (27.8421, -64.5659) -> (44.9421, -64.5659)
  line L71 (44.9421, -64.5659) -> (44.9421, -80.8159)
  arc A3 (-19.3579, 5.1341) -> (-24.3579, 0.1341) centre (-19.3579, 0.1341) ccw
  line L72 (-24.3579, 0.1341) -> (-24.3579, -84.0159)
  arc A4 (-24.3579, -84.0159) -> (-19.3579, -89.0159) centre (-19.3579, -84.0159) ccw
  line L73 (-19.3579, -89.0159) -> (92.1421, -89.0159)
  arc A5 (92.1421, -89.0159) -> (97.1421, -84.0159) centre (92.1421, -84.0159) ccw
  line L74 (97.1421, -84.0159) -> (97.1421, -62.4409)
  line L75 (97.1421, -62.4409) -> (75.3921, -62.4409)
  arc A6 (69.3921, -56.4409) -> (75.3921, -62.4409) centre (75.3921, -56.4409) ccw
  line L76 (69.3921, -56.4409) -> (69.3921, 5.1341)
  line L77 (69.3921, 5.1341) -> (-19.3579, 5.1341)
  line L78 (49.8421, -52.1909) -> (80.3921, -52.1909) construction
  line L79 (80.3921, -80.8159) -> (80.3921, -52.1909) construction
  circle A7 centre (-20.6579, -85.3159) radius 1.625
  circle A8 centre (-20.6579, 1.4341) radius 1.625
  circle A9 centre (93.4421, -85.3159) radius 1.625
  circle A10 centre (93.4421, 1.4341) radius 2.5
  dimension "d96" = 4.85
  dimension "d97" = 6.25
  constraint concentric A1 A2
  constraint midpoint L59 L79.start
  constraint perpendicular L0 L79
  constraint midpoint L13 L78.start
  constraint perpendicular L78 L79
  measures "d96" diameter of A1
  measures "d97" diameter of A2
extrude "Extrude16" cut sketch "Sketch5" against normal blind 3.5 contours A1 bodies 2
extrude "Extrude17" cut sketch "Sketch5" against normal blind 13.5 from surface at -3.5 contours A1 | A2 bodies 2
sketch "Sketch6" plane through (0, 0, -2) normal (0, 0, -1) x (1, 0, 0)
  line L0 (21.6579, 2.4341) -> (-94.4421, 2.4341)
  line L1 (-94.4421, 2.4341) -> (-94.4421, -86.3159)
  line L2 (-94.4421, -86.3159) -> (21.6579, -86.3159)
  line L3 (21.6579, -86.3159) -> (21.6579, 2.4341)
  circle A0 centre (-83.1073, -7.8043) radius 6.375
  line L4 (-94.4421, -41.9409) -> (-57.337, -41.9409) construction
  line L5 (-36.3921, 2.4341) -> (-36.3921, -15.5353) construction
  circle A1 centre (10.323, -7.8043) radius 6.375
  circle A2 centre (-83.1073, -76.0776) radius 6.375
  circle A3 centre (10.323, -76.0776) radius 6.375
  dimension "d103" = 12.75
  constraint midpoint L1 L4.start
  constraint perpendicular L1 L4
  constraint midpoint L0 L5.start
  constraint perpendicular L0 L5
  constraint symmetric A0 L5 A1
  constraint symmetric A0 L4 A2
  constraint symmetric L4 A1 A3
  measures "d103" diameter of A0
extrude "Extrude18" cut sketch "Sketch6" against normal blind 0.8 contours A0 | A1 | A2 | A3 bodies 1
equation "d1 = 16.5 mm + Tolerances"
equation "d2 = 15.65 mm + Tolerances"
equation "Tolerances = 0.6 mm"
equation "d34 = 0.6 mm - 1 mm"
equation "d36 = SwitchFitOffset"
equation "d37 = SwitchFitOffset"
equation "SwitchFitOffset = ( 1.25 / 2 ) * 1 mm"
equation "d39 = SwitchFitOffset"
equation "d40 = SwitchFitOffset"
equation "d41 = SwitchFitOffset"
equation "d42 = SwitchFitOffset"
equation "d43 = SwitchFitOffset"
equation "d44 = SwitchFitOffset"
equation "d45 = SwitchFitOffset"
equation "d46 = SwitchFitOffset"
equation "d47 = SwitchFitOffset"
equation "d48 = SwitchFitOffset"
equation "d49 = SwitchFitOffset"
equation "d50 = SwitchFitOffset"
equation "d51 = SwitchFitOffset"
equation "d52 = SwitchFitOffset"
equation "d53 = SwitchFitOffset"
equation "d54 = SwitchFitOffset"
equation "d60 = -Tolerances / 2"
equation "d62 = -Tolerances / 2"
equation "d64 = -Tolerances / 2"
equation "d66 = -Tolerances / 2"
named bodies: "Case", "Key Insert"
